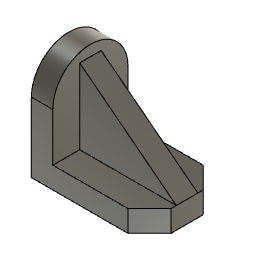
object  A1 (Autodesk Fusion 360 design; units mm, degrees)
Autodesk Fusion 360 part; units mm, degrees
sketch "the horizontal part sketch" plane through (0, 0, 0) normal (0, 0, 1) x (1, 0, 0)
  line L0 (-33, 21) -> (33, 21)
  line L1 (33, 21) -> (33, -21)
  line L2 (33, -21) -> (-33, -21)
  line L3 (-33, -21) -> (-33, 21)
  line L4 (-33, 21) -> (33, -21) construction
  line L5 (33, 21) -> (-33, -21) construction
  dimension "d1" = 66
  dimension "d2" = 42
  constraint horizontal L0
  constraint perpendicular L0 L1
  constraint parallel L0 L2
  constraint parallel L1 L3
  constraint coincident L4 origin
  constraint coincident L5 origin
  measures "d1" distance of L0.start L0.end
  measures "d2" distance of L0.end L1.end
extrude "Extrude1" add sketch "the horizontal part sketch" along normal blind 12 makes body 1
sketch "the vertical part sketch" plane through (0, 0, 12) normal (0, 0, 1) x (-1, 0, 0)
  line L0 (33, 21) -> (-33, 21)
  line L1 (-33, 21) -> (-33, -21)
  line L2 (-33, -21) -> (33, -21)
  line L3 (33, -21) -> (33, 21)
  line L4 (33, -21) -> (21, -21)
  line L5 (21, -21) -> (21, 21)
  line L6 (21, 21) -> (33, 21)
  line L7 (33, 21) -> (33, -21)
  dimension "d5" = 12
  constraint horizontal L4
  constraint vertical L5
  constraint horizontal L6
  constraint vertical L7
  constraint coincident L0 L5.end
  constraint coincident L2.end L3.start
  measures "d5" distance of L2.end L4.end
extrude "Extrude2" add sketch "the vertical part sketch" along normal blind 48 contours L0 L2 L3 L4 L5 L6 L7 bodies 1
fillet "Fillet1" radius 21 1 edges at (-27, -21, 60) on bodies 1
fillet "Fillet2" radius 21 1 edges at (-27, 21, 60) on bodies 1
chamfer "Chamfer1" distance 12 angle 45 1 edges at (33, 21, 6) on bodies 1
chamfer "Chamfer2" distance 12 angle 45 1 edges at (33, -21, 6) on bodies 1
sketch "triangle sketch" plane through (0, 0, 0) normal (0, 1, 0) x (1, 0, 0)
  line L0 (-21, -54) -> (-21, -12)
  line L1 (-21, -12) -> (33, -12)
  line L2 (33, -12) -> (-21, -54)
  dimension "d14" = 42
  dimension "d15" = 54
  constraint vertical L0
  constraint perpendicular L0 L1
  measures "d14" distance of L0.start L0.end
  measures "d15" distance of L0.end L1.end
extrude "Extrude3" add sketch "triangle sketch" along normal mid plane 12 bodies 1
copy_body "Body->Comp1" bodies 1 removing the originals makes body 2 in component "object A1"
component "object A1" placed x (1, 0, 0) y (0, 1, 0) z (0, 0, 1) at (0, 0, 0)
equation "d6 = 60 mm - 12 mm"
equation "d15 = 66 mm - 12 mm"
named bodies: "object A1"
